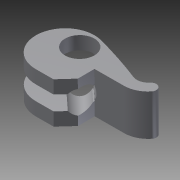
# Autodesk Inventor part: cam
Saved by Autodesk Inventor 2012 (Build 160160000, 160)
## iProperties
Created: 2012-01-06
Part Number: cam
Material: Default
Document SubType Name: Modeling
Designer: Kennell
Density: 1 g/cm^3
Author: Kennell
Autodesk Inventor part; units mm, degrees
ref_plane "YZ Plane" through (0, 0, 0) normal (1, 0, 0) x (0, 1, 0)
ref_plane "XZ Plane" through (0, 0, 0) normal (0, 1, 0) x (-1, 0, 0)
sketch "Sketch1" plane through (0, 0, 0) normal (0, 0, 1) x (1, 0, 0)
  line L0 (0, -10) -> (10, -10)
  line L1 (10, -10) -> (10, 0)
  line L2 (10, 0) -> (20.073, 0)
  arc A0 (20.073, 0) -> (26.4599, 3.0109) centre (20.073, 8.2794) ccw
  arc A1 (26.4599, 3.0109) -> (23.6035, 5.3671) centre (25.0317, 4.189) ccw
  arc A2 (19.1208, 4.2044) -> (23.6035, 5.3671) centre (20.5602, 7.8775) ccw
  arc A3 (19.1208, 4.2044) -> (2.6102, 9.6533) centre (-38.895, -143.8482) ccw
  arc A4 (2.6102, 9.6533) -> (0, -10) centre (0, 0) ccw
  dimension "d2" = 10
  dimension "d3" = 10
  dimension "d4" = 8.2794
  dimension "d5" = 10.073
  dimension "d6" = 159.0138
  dimension "d7" = 4.9587
  dimension "d8" = 4.189
  dimension "d9" = 7.8775
  dimension "d10" = 0.4872
  dimension "d11" = 10
  constraints: 10 point on circle, 6 end point, 6 tangent, 5 centre point, 2 perpendicular, 1 coincident, 1 horizontal
  measures "d2" distance of L0.start L0.end
  measures "d3" distance of L0.end L1.end
  measures "d4" distance of L2.end A0.centre
  measures "d5" distance of L1.end L2.end
  measures "d6" radius of A3
  measures "d7" horizontal distance of L2.end A1.centre
  measures "d8" vertical distance of A1.centre L2.end
  measures "d9" vertical distance of L2.end A2.centre
  measures "d10" horizontal distance of A2.centre L2.end
  measures "d11" radius of A4
extrude "Extrusion1" add sketch "Sketch1" along normal blind 14
hole "Hole1" at (1, 4, 14) direction (0, 0, -1) diameter 10 end through all
sketch "Sketch2" plane through (0, 0, 14) normal (0, 0, 1) x (1, 0, 0)
  line L0 (10, -10) -> (0, -10) projected
  line L1 (10, 0) -> (10, -10) projected
  line L2 (10, -5.7007) -> (6, -10)
  line L3 (10, -10) -> (10, -5.7007)
  constraints: 4 end point, 2 point on line, 1 collinear
extrude "Extrusion2" cut sketch "Sketch2" against normal through all
ref_plane "Work Plane1" through (10, -5.7007, 14) normal (0.7321313, -0.6811636, 0) x (0, 0, -1)
sketch "Sketch3" plane through (10, -5.7007, 14) normal (0.7321313, -0.6811636, 0) x (0, 0, -1)
  line L0 (14, 4.1737) -> (0, 4.1737) projected
  line L1 (0, 4.1737) -> (0, 0) projected
  line L2 (14, 0) -> (14, 4.1737) projected
  line L3 (14, 6.2075) -> (0, 6.2075) projected
  line L4 (14, 11.035) -> (0, 11.035) projected
  line L5 (14, 4.1737) -> (14, 11.035) projected
  line L6 (0, 11.035) -> (0, 4.1737) projected
  line L7 (14, -11.2349) -> (0, -11.2349) projected
  line L8 (14, -4.0283) -> (0, -4.0283) projected
  line L9 (4.5, 4.1737) -> (9.5, 4.1737)
  line L10 (9.5, 4.1737) -> (9.5, -15.8263)
  line L11 (9.5, -15.8263) -> (4.5, -15.8263)
  line L12 (4.5, -15.8263) -> (4.5, 4.1737)
  circle A0 centre (7, 0.6737) radius 4
  point P0 (14, -2.638)
  point P1 (7, -15.8263)
  point P2 (7, -11.2349)
  point P3 (7, 3.305)
  point P4 (7, 4.1737)
  dimension "d27" = 5
  dimension "d28" = 20
  dimension "d31" = 8
  dimension "d32" = 3.5
  constraints: 8 end point, 3 midpoint, 2 parallel, 2 vertical alignment, 1 centre point, 1 horizontal, 1 perpendicular, 1 point on line
  measures "d27" distance of L10.end L11.end
  measures "d28" distance of L9.end L10.end
  measures "d31" diameter of A0
  measures "d32" distance from line of L0 A0.centre
extrude "Extrusion3" cut sketch "Sketch3" against normal through all contours L10 A0 L0 | A0 L10 L12 L0 | A0 L12 L0 | L10 L8 L12 A0 | L10 L7 L12 L8 | L10 L11 L12 L7
extrude "Extrusion4" cut sketch "Sketch3" against normal blind 14 contours A0 L10 L12 L0 | L0 A0 | A0 L10 | L12 A0
hole "Hole2" at (-0.1315, 9.4262, 7.0072) direction (0.6811636, 0.7321313, 0) diameter 5 end through all
body "Solid1"
